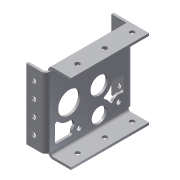
# Autodesk Inventor part: GearboxPlate
Saved by Autodesk Inventor 2013 SP1 (Build 170176100, 176)
## iProperties
Created: 2013-12-02
Part Number: GearboxPlate
Material: Aluminum 6061
Document SubType Name: Sheet Metal
Designer: robotics
Density: 2.71 g/cm^3
Sheet Metal Rule: 3mm Aluminum
Author: robotics
Autodesk Inventor part; units mm, degrees
ref_plane "YZ Plane" through (0, 0, 0) normal (1, 0, 0) x (0, 1, 0)
ref_plane "XZ Plane" through (0, 0, 0) normal (0, 1, 0) x (-1, 0, 0)
ref_plane "XY Plane" through (0, 0, 0) normal (0, 0, 1) x (1, 0, 0)
sketch "Sketch1" plane through (0, 0, 0) normal (1, 0, 0) x (0, 1, 0)
  line L0 (-50, 45) -> (50, 45)
  line L1 (50, 45) -> (50, -45)
  line L2 (50, -45) -> (-50, -45)
  line L3 (-50, -45) -> (-50, 45)
  point P0 (0, 0)
  dimension "d0" = 100
  dimension "d35" = 90
  dimension "d36" = 50
  dimension "d37" = 45
  measures "d0" distance of L0.start L0.end
  measures "d35" distance of L0.end L1.end
  measures "d36" distance from line of L1 point (0, 0)
  measures "d37" distance from line of L0 point (0, 0)
extrude "Plate1" add sketch "Sketch1" along normal blind 3
sketch "Sketch2" plane through (-3, 53, -45) normal (0, 1, 0) x (-1, 0, 0)
  line L0 (0, 90) -> (0, 0)
  line L1 (0, 0) -> (19, 0)
  line L2 (19, 0) -> (19, 90)
  line L3 (19, 90) -> (0, 90)
  constraints: 6 end point, 1 horizontal, 1 perpendicular, 1 vertical
edge flange "Flange1" height 25 angle 90 thickness 3 bend radius 3 thickness toward (0, 1, 0) relief straight relief width 3 relief depth 1.5 corner gap 3 corner form 0 edges at (0, 50, 0) (0, -50, 0) wall of the first edge with corners at (-3, 53, 45) (-3, 53, -45) (-22, 53, -45) (-22, 53, 45)
bend "Bend1"
corner "Corner1"
sketch "Sketch3" plane through (6, -50, 48) normal (0, 0, 1) x (1, 0, 0)
  line L0 (0, 100) -> (0, 0)
  line L1 (0, 0) -> (23.4696, 0)
  line L2 (23.4696, 0) -> (23.4696, 100)
  line L3 (23.4696, 100) -> (0, 100)
  constraints: 6 end point, 1 horizontal, 1 perpendicular, 1 vertical
edge flange "Flange2" height 29.4696 angle 90 thickness 3 bend radius 3 thickness toward (0, 0, 1) relief straight relief width 3 relief depth 1.5 corner gap 3 corner form 0 edges at (3, 0, 45) (3, 0, -45) wall of the first edge with corners at (6, 50, 48) (6, -50, 48) (29.4696, -50, 48) (29.4696, 50, 48)
bend "Bend2"
corner "Corner2"
sketch "Sketch4" plane through (3, 0, 0) normal (1, 0, 0) x (0, 0, -1)
  line L0 (-45, 50) -> (45, 50) projected
  line L1 (-45, -50) -> (-45, 50) projected
  line L2 (45, -50) -> (-45, -50) projected
  line L3 (45, 50) -> (45, -50) projected
  circle A0 centre (-31.5962, 12.4637) radius 7.62 construction
  circle A1 centre (1.5, 12.4637) radius 12.7 construction
  circle A2 centre (34.5962, 12.4637) radius 7.62 construction
  circle A3 centre (1.5, -25.7125) radius 25.4 construction
  circle A4 centre (1.5, 12.4637) radius 25.4 construction
  line L4 (26.9762, 12.4637) -> (26.9, 12.4637) construction
  line L5 (-23.9762, 12.4637) -> (-23.9, 12.4637) construction
  line L6 (1.5, -0.3125) -> (1.5, -0.2363) construction
  line L7 (-33.5, -12.8649) -> (-29.6924, 37.7923) construction
  line L8 (36.5, -12.8649) -> (32.6924, 37.7923) construction
  point P0 (0, 0)
  dimension "d24" = 25.4
  dimension "d25" = 15.24
  dimension "d27" = 50.8
  dimension "d23" = 0.0762
  dimension "d26" = 50.8
  dimension "d34" = 66.1924
  dimension "d38" = 24.2875
  dimension "d40" = 46.5
  dimension "d41" = 43.5
  dimension "d42" = 50.8
  dimension "d45" = 70
  constraints: 10 end point, 5 horizontal alignment, 3 coincident, 3 equal length, 3 vertical alignment, 2 horizontal, 2 line through centre, 2 midpoint, 2 point on circle, 2 vertical, 1 centre point, 8 other
  measures "d23" distance of L6.start L6.end
  measures "d26" diameter of A4
  measures "d34" distance of point (34.596, 12.464) point (-31.596, 12.464)
  measures "d38" distance from line of L2 point (1.5, -25.712)
  measures "d40" distance from line of L1 point (1.5, 12.464)
  measures "d41" distance from line of L3 point (1.5, 12.464)
  measures "d42" distance of L7.start L7.end
  measures "d45" distance of L8.start L7.start
sketch "Sketch5" plane through (3, 0, 0) normal (1, 0, 0) x (0, 0, -1)
  circle A0 centre (-31.5962, 12.4637) radius 9.525
  circle A1 centre (34.5962, 12.4637) radius 9.525
  circle A2 centre (1.5, 12.4637) radius 11.1125
  circle A3 centre (1.5, -25.7125) radius 14.2875
  line L0 (-33.5, -12.8649) -> (-29.6924, 37.7923) construction
  line L1 (36.5, -12.8649) -> (32.6924, 37.7923) construction
  circle A4 centre (-29.6924, 37.7923) radius 3
  circle A5 centre (32.6924, 37.7923) radius 3
  circle A6 centre (36.5, -12.8649) radius 3
  circle A7 centre (-33.5, -12.8649) radius 3
  point P0 (0, 0)
  dimension "d28" = 19.05
  dimension "d30" = 22.225
  dimension "d31" = 28.575
  dimension "d44" = 6
  constraints: 8 centre point, 8 coincident, 4 equal radius
  measures "d28" diameter of A0
  measures "d30" diameter of A2
  measures "d31" diameter of A3
  measures "d44" diameter of A5
extrude "Cut1" cut sketch "Sketch5" against normal blind 3
sketch "Sketch7" plane through (29.4696, -50, 51) normal (0, 0, 1) x (1, 0, 0)
  line L0 (-23.4696, 100) -> (-23.4696, 0) projected
  line L1 (0, 100) -> (0, 0) projected
  line L2 (-23.4696, 100) -> (0, 100) projected
  circle A0 centre (-11.7348, 90) radius 3
  circle A1 centre (-11.7348, 55) radius 3
  circle A2 centre (-11.7348, 20) radius 3
  point P0 (-29.4696, 50)
  dimension "d72" = 6
  dimension "d74" = 11.7348
  dimension "d75" = 11.7348
  dimension "d76" = 10
  dimension "d79" = 35
  constraints: 3 centre point, 1 vertical, 4 other
  measures "d72" diameter of A0
  measures "d74" distance from line of L1 A0.centre
  measures "d75" distance from line of L0 A0.centre
  measures "d76" distance from line of L2 A0.centre
  measures "d79" distance of A0.centre A1.centre
extrude "Cut3" cut sketch "Sketch7" against normal through all
sketch "Sketch8" plane through (-22, 56, 45) normal (0, 1, 0) x (1, 0, 0)
  line L0 (19, 0) -> (19, 90) projected
  line L1 (0, 0) -> (0, 90) projected
  line L2 (19, 0) -> (0, 0) projected
  circle A0 centre (9.5, 15) radius 3
  circle A1 centre (9.5, 35) radius 3
  circle A2 centre (9.5, 55) radius 3
  circle A3 centre (9.5, 75) radius 3
  point P0 (22, 45)
  dimension "d86" = 6
  dimension "d88" = 9.5
  dimension "d89" = 9.5
  dimension "d90" = 15
  dimension "d93" = 20
  constraints: 4 centre point, 1 vertical, 6 other
  measures "d86" diameter of A0
  measures "d88" distance from line of L0 A0.centre
  measures "d89" distance from line of L1 A0.centre
  measures "d90" distance from line of L2 A0.centre
  measures "d93" distance of A0.centre A1.centre
extrude "Cut4" cut sketch "Sketch8" against normal through all
sketch "Sketch9" plane through (0, 0, 0) normal (-1, 0, 0) x (0, 0, 1)
  circle A0 centre (-1.5, 12.4637) radius 11.1125 projected
  circle A1 centre (-32.6924, 37.7923) radius 3 projected
  circle A2 centre (-34.5962, 12.4637) radius 9.525 projected
  line L0 (45, 50) -> (-45, 50) projected
  arc A3 (-20.715, 19.4163) -> (-27.9683, 26.5028) centre (-34.5962, 12.4637) ccw
  arc A4 (-28.1286, 30.0352) -> (-24.3769, 41.235) centre (-32.6924, 37.7923) ccw
  arc A5 (-5.9768, 28.9802) -> (-17.1032, 19.4907) centre (-1.5, 12.4637) ccw
  line L1 (-6.5, 44) -> (-22.529, 44)
  arc A6 (-28.1286, 30.0352) -> (-27.9683, 26.5028) centre (-27.1145, 28.3114) ccw
  arc A7 (-22.529, 44) -> (-24.3769, 41.235) centre (-22.529, 42) ccw
  arc A8 (-20.715, 19.4163) -> (-17.1032, 19.4907) centre (-18.9268, 20.3119) ccw
  circle A9 centre (-36.5, -12.8649) radius 3 projected
  circle A10 centre (-1.5, -25.7125) radius 14.2875 projected
  line L2 (-45, 50) -> (-45, -50) projected
  line L3 (-45, -50) -> (45, -50) projected
  line L4 (-4.5, 30.9106) -> (-4.5, 42)
  arc A11 (-4.5, 42) -> (-6.5, 44) centre (-6.5, 42) ccw
  arc A12 (-5.9768, 28.9802) -> (-4.5, 30.9106) centre (-6.5, 30.9106) ccw
  line L5 (-1.5, 12.4637) -> (-1.5, -25.7125)
  arc A13 (-21.6278, -23.1723) -> (-15.3483, -40.5384) centre (-1.5, -25.7125) ccw
  arc A14 (-36.9091, -21.8555) -> (-30.3842, -19.4676) centre (-36.5, -12.8649) ccw
  line L6 (-39, -23.8535) -> (-39, -42)
  line L7 (-16.7135, -44) -> (-37, -44)
  arc A15 (-39, -42) -> (-37, -44) centre (-37, -42) ccw
  arc A16 (-16.7135, -44) -> (-15.3483, -40.5384) centre (-16.7135, -42) ccw
  arc A17 (-36.9091, -21.8555) -> (-39, -23.8535) centre (-37, -23.8535) ccw
  line L8 (-28.3359, -19.0574) -> (-22.9229, -21.0444)
  arc A18 (-28.3359, -19.0574) -> (-30.3842, -19.4676) centre (-29.0251, -20.9349) ccw
  arc A19 (-21.6278, -23.1723) -> (-22.9229, -21.0444) centre (-23.6121, -22.9219) ccw
  arc A20 (-27.5648, -11.7869) -> (-30.828, -5.8772) centre (-36.5, -12.8649) ccw
  arc A21 (-8.7645, -6.7702) -> (-18.4911, -14.6272) centre (-1.5, -25.7125) ccw
  arc A22 (-17.1032, 5.4367) -> (-8.6455, -3.0855) centre (-1.5, 12.4637) ccw
  arc A23 (-30.1414, -2.4084) -> (-20.715, 5.5111) centre (-34.5962, 12.4637) ccw
  line L9 (-26.2684, -13.4249) -> (-20.8554, -15.4119)
  arc A24 (-27.5648, -11.7869) -> (-26.2684, -13.4249) centre (-25.5792, -11.5474) ccw
  arc A25 (-30.1414, -2.4084) -> (-30.828, -5.8772) centre (-29.5675, -4.3243) ccw
  arc A26 (-17.1032, 5.4367) -> (-20.715, 5.5111) centre (-18.9268, 4.6155) ccw
  arc A27 (-8.7645, -6.7702) -> (-8.6455, -3.0855) centre (-9.4807, -4.9028) ccw
  arc A28 (-20.8554, -15.4119) -> (-18.4911, -14.6272) centre (-20.1662, -13.5344) ccw
  arc A29 (24.9683, 26.5028) -> (17.715, 19.4163) centre (31.5962, 12.4637) ccw
  arc A30 (21.3769, 41.235) -> (25.1286, 30.0352) centre (29.6924, 37.7923) ccw
  arc A31 (14.1032, 19.4907) -> (2.9768, 28.9802) centre (-1.5, 12.4637) ccw
  line L10 (3.5, 44) -> (19.529, 44)
  arc A32 (24.9683, 26.5028) -> (25.1286, 30.0352) centre (24.1145, 28.3114) ccw
  arc A33 (21.3769, 41.235) -> (19.529, 44) centre (19.529, 42) ccw
  arc A34 (14.1032, 19.4907) -> (17.715, 19.4163) centre (15.9268, 20.3119) ccw
  line L11 (1.5, 30.9106) -> (1.5, 42)
  arc A35 (3.5, 44) -> (1.5, 42) centre (3.5, 42) ccw
  arc A36 (1.5, 30.9106) -> (2.9768, 28.9802) centre (3.5, 30.9106) ccw
  arc A37 (12.3483, -40.5384) -> (18.6278, -23.1723) centre (-1.5, -25.7125) ccw
  arc A38 (27.3842, -19.4676) -> (33.9091, -21.8555) centre (33.5, -12.8649) ccw
  line L12 (36, -23.8535) -> (36, -42)
  line L13 (13.7135, -44) -> (34, -44)
  arc A39 (34, -44) -> (36, -42) centre (34, -42) ccw
  arc A40 (12.3483, -40.5384) -> (13.7135, -44) centre (13.7135, -42) ccw
  arc A41 (36, -23.8535) -> (33.9091, -21.8555) centre (34, -23.8535) ccw
  line L14 (25.3359, -19.0574) -> (19.9229, -21.0444)
  arc A42 (27.3842, -19.4676) -> (25.3359, -19.0574) centre (26.0251, -20.9349) ccw
  arc A43 (19.9229, -21.0444) -> (18.6278, -23.1723) centre (20.6121, -22.9219) ccw
  arc A44 (27.828, -5.8772) -> (24.5648, -11.7869) centre (33.5, -12.8649) ccw
  arc A45 (15.4911, -14.6272) -> (5.7645, -6.7702) centre (-1.5, -25.7125) ccw
  arc A46 (5.6455, -3.0855) -> (14.1032, 5.4367) centre (-1.5, 12.4637) ccw
  arc A47 (17.715, 5.5111) -> (27.1414, -2.4084) centre (31.5962, 12.4637) ccw
  line L15 (23.2684, -13.4249) -> (17.8554, -15.4119)
  arc A48 (23.2684, -13.4249) -> (24.5648, -11.7869) centre (22.5792, -11.5474) ccw
  arc A49 (27.828, -5.8772) -> (27.1414, -2.4084) centre (26.5675, -4.3243) ccw
  arc A50 (17.715, 5.5111) -> (14.1032, 5.4367) centre (15.9268, 4.6155) ccw
  arc A51 (5.6455, -3.0855) -> (5.7645, -6.7702) centre (6.4807, -4.9028) ccw
  arc A52 (15.4911, -14.6272) -> (17.8554, -15.4119) centre (17.1662, -13.5344) ccw
  point P0 (0, 0)
  point P1 (-26.176, 44)
  dimension "d100" = 6
  dimension "d101" = 6
  dimension "d102" = 6
  dimension "d103" = 6
  dimension "d105" = 2
  dimension "d108" = 6
  dimension "d109" = 6
  dimension "d110" = 3
  dimension "d111" = 6
  dimension "d112" = 6
  dimension "d113" = 3
  dimension "d114" = 6
  constraints: 97 point on circle, 50 symmetric about line, 48 centre point, 30 tangent, 26 end point, 19 equal radius, 13 coincident, 3 parallel, 2 perpendicular, 1 horizontal, 1 point on line, 24 other
  measures "d100" radial gap between concentric circles of A2 A3
  measures "d101" radial gap between concentric circles of A0 A5
  measures "d102" radial gap between concentric circles of A1 A4
  measures "d103" distance between parallel lines of L0 L1
  measures "d105" radius of A7
  measures "d108" diameter of L4 L5
  measures "d109" radial gap between concentric circles of A10 A13
  measures "d110" distance from line of L5.end L8
  measures "d111" distance between parallel lines of L3 L7
  measures "d112" distance between parallel lines of L2 L6
  measures "d113" distance from line of A9.centre L8
  measures "d114" distance between parallel lines of L9 L8
extrude "Cut5" cut sketch "Sketch9" against normal blind 3 contours A3 A6 A4 A7 L1 A11 L4 A12 A5 A8 | A13 A16 L7 A15 L6 A17 A14 A18 L8 A19 | A20 A25 A23 A26 A22 A27 A21 A28 L9 A24 | A29 A34 A31 A36 L11 A35 L10 A33 A30 A32 | A37 A43 L14 A42 A38 A41 L12 A39 L13 A40 | A44 A48 L15 A52 A45 A51 A46 A50 A47 A49
equation "\"d32\" = Thickness"
equation "\"d3\" = BendReliefWidth"
equation "\"d4\" = BendReliefDepth"
equation "\"d5\" = MinimumRemnant"
equation "\"d6\" = BendRadius"
equation "\"d9\" = BendRadius"
equation "\"d10\" = CornerReliefSize"
equation "\"d11\" = GapSize"
equation "\"d12\" = JacobiRadiusSize"
equation "\"d13\" = BendReliefWidth"
equation "\"d14\" = BendReliefDepth"
equation "\"d15\" = MinimumRemnant"
equation "\"d16\" = BendRadius"
equation "\"d19\" = BendRadius"
equation "\"d20\" = CornerReliefSize"
equation "\"d21\" = GapSize"
equation "\"d22\" = JacobiRadiusSize"
equation "\"d36\" = 0.5 * d0"
equation "\"d37\" = 0.5 * d35"
equation "\"BendRadius\" = Thickness"
equation "\"BendReliefWidth\" = Thickness"
equation "\"BendReliefDepth\" = 0.5 * Thickness"
equation "\"CornerReliefSize\" = 4 * Thickness"
equation "\"MinimumRemnant\" = 2 * Thickness"
equation "\"TransitionRadius\" = BendRadius"
equation "\"JacobiRadiusSize\" = BendRadius"
equation "\"GapSize\" = Thickness"
equation "\"d2\" = BendRadius"
equation "\"Thickness\" = 3"
body "Solid1"
